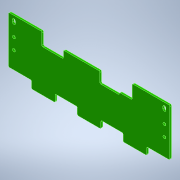
# Autodesk Inventor part: USB_MAIN_PCB
Saved by Autodesk Inventor 2021 (Build 250183000, 183)
## iProperties
Created: 2020-06-13
Part Number: USB_MAIN_PCB
Material: Generic
Document SubType Name: Modeling
Designer: Viktor Lindström
Density: 1 g/cm^3
Appearance: Default
Author: Viktor Lindström
Autodesk Inventor part; units mm, degrees
ref_plane "YZ Plane" through (0, 0, 0) normal (1, 0, 0) x (0, 1, 0)
ref_plane "XZ Plane" through (0, 0, 0) normal (0, 1, 0) x (-1, 0, 0)
ref_plane "XY Plane" through (0, 0, 0) normal (0, 0, 1) x (1, 0, 0)
sketch "Sketch1" plane through (0, 0, 0) normal (0, 0, 1) x (1, 0, 0)
  line L0 (-71, -23) -> (71, -23)
  line L1 (71, -23) -> (71, 23)
  line L2 (71, 23) -> (-71, 23)
  line L3 (-71, 23) -> (-71, -23)
  line L4 (-71, -23) -> (71, 23) construction
  line L5 (71, -23) -> (-71, 23) construction
  point P0 (0, 0)
  dimension "d2" = 142
  dimension "d3" = 46
  constraints: 12 end point, 2 midpoint, 2 parallel, 1 horizontal, 1 perpendicular
  measures "d2" distance of L1.end L2.end
  measures "d3" distance of L2.end L0.start
extrude "Extrusion1" add sketch "Sketch1" along normal blind 1.6
sketch "Sketch2" plane through (0, 0, 1.6) normal (0, 0, 1) x (1, 0, 0)
  line L0 (71, -23) -> (71, 23) projected
  line L1 (71, 23) -> (-71, 23) projected
  line L2 (-71, 23) -> (-71, -23) projected
  line L3 (-71, -23) -> (71, -23) projected
  line L4 (28, 23) -> (10, 23)
  line L5 (10, 23) -> (10, 13)
  line L6 (10, 13) -> (28, 13)
  line L7 (28, 13) -> (28, 23)
  point P0 (0, 0)
  dimension "d4" = 43
  dimension "d5" = 18
  dimension "d6" = 10
  constraints: 8 end point, 2 parallel, 1 horizontal, 1 perpendicular, 1 point on line
  measures "d4" distance between parallel lines of L7 L0
  measures "d5" distance between parallel lines of L7 L5
  measures "d6" distance between parallel lines of L1 L6
extrude "Extrusion2" cut sketch "Sketch2" against normal through all contours L7 L6 L5 L1
sketch "Sketch3" plane through (0, 0, 1.6) normal (0, 0, 1) x (1, 0, 0)
  line L0 (10, 13) -> (10, 23) construction
  line L1 (10, 23) -> (-71, 23) construction
  line L2 (-71, 23) -> (-71, -23) construction
  line L3 (-71, -23) -> (71, -23) construction
  line L4 (71, -23) -> (71, 23) construction
  line L5 (71, 23) -> (28, 23) construction
  line L6 (28, 23) -> (28, 13) construction
  line L7 (28, 13) -> (10, 13) construction
  line L8 (71, -23) -> (71, 23) projected
  line L9 (71, -23) -> (53.584, -23)
  line L10 (53.584, -23) -> (53.584, -16)
  line L11 (53.584, -16) -> (71, -16)
  line L12 (71, -16) -> (71, -23)
  line L13 (31.584, -23) -> (11, -23)
  line L14 (11, -23) -> (11, -16)
  line L15 (11, -16) -> (31.584, -16)
  line L16 (31.584, -16) -> (31.584, -23)
  line L17 (-71, -23) -> (71, -23) projected
  line L18 (-11, -23) -> (-31.584, -23)
  line L19 (-31.584, -23) -> (-31.584, -16)
  line L20 (-31.584, -16) -> (-11, -16)
  line L21 (-11, -16) -> (-11, -23)
  line L22 (-71, -23) -> (-53.584, -23)
  line L23 (-53.584, -23) -> (-53.584, -16)
  line L24 (-53.584, -16) -> (-71, -16)
  line L25 (-71, -16) -> (-71, -23)
  point P0 (0, 0)
  point P1 (3, -23)
  point P2 (-3, -23)
  dimension "d10" = 7
  dimension "d11" = 7
  dimension "d15" = 7
  dimension "d62" = 22
  dimension "d63" = 22
  dimension "d82" = 53.584
  dimension "d83" = 53.584
  dimension "d84" = 22
  dimension "d85" = 11
  constraints: 32 end point, 8 parallel, 4 horizontal, 4 perpendicular, 4 point on line
  measures "d10" distance between parallel lines of L22 L24
  measures "d11" distance between parallel lines of L9 L11
  measures "d15" distance between parallel lines of L13 L15
  measures "d62" distance between parallel lines of L19 L23
  measures "d63" distance between parallel lines of L10 L16
  measures "d82" distance from line of point (0, 0) L10
  measures "d83" distance from line of point (0, 0) L23
  measures "d84" distance between parallel lines of L21 L14
  measures "d85" distance from line of point (0, 0) L14
extrude "Extrusion3" cut sketch "Sketch3" against normal through all
sketch "Sketch5" plane through (0, 0, 1.6) normal (0, 0, 1) x (1, 0, 0)
  line L0 (-71, -16) -> (-53.584, -16) construction
  line L1 (53.584, -16) -> (71, -16) projected
  line L2 (-71, 23) -> (-71, -16) projected
  line L3 (-71, -16) -> (-75, -16)
  line L4 (-75, -16) -> (-75, 23)
  line L5 (-75, 23) -> (-71, 23)
  line L6 (-71, 23) -> (-71, -16)
  line L7 (71, 20) -> (71, -16)
  line L8 (0, -33.4899) -> (0, 38.4899) projected
  line L9 (71, 23) -> (71, -16)
  line L10 (71, -16) -> (75, -16)
  line L11 (75, -16) -> (75, 23)
  line L12 (75, 23) -> (71, 23)
  line L13 (71, 23) -> (71, -16)
  point P0 (0, 0)
  point P1 (71, 23)
  point P2 (71, 23)
  point P3 (-71, 22.2558)
  dimension "d32" = 75
  constraints: 20 end point, 4 symmetric about line, 2 parallel, 1 horizontal, 1 perpendicular, 1 point on line
  measures "d32" distance from line of L4 point (0, 0)
extrude "Extrusion5" add sketch "Sketch5" against normal up to surface (1.6 mm away)
sketch "Sketch6" plane through (0, 0, 0) normal (0, 0, -1) x (-1, 0, 0)
  circle A0 centre (70, 10.5) radius 1.375
  circle A1 centre (70, 0) radius 1.375
  line L0 (75, -16) -> (75, 23) construction
  line L1 (-10, 23) -> (75, 23) construction
  line L2 (0, -33.4899) -> (0, 38.4899) projected
  circle A2 centre (-70, 10.5) radius 1.375
  circle A3 centre (-70, 0) radius 1.375
  point P0 (0, 0)
  point P1 (-75, -16)
  point P2 (71, 23)
  dimension "d35" = 2.75
  dimension "d36" = 2.75
  dimension "d37" = 5
  dimension "d38" = 5
  dimension "d39" = 12.5
  dimension "d40" = 10.5
  constraints: 4 centre point, 3 symmetric about line, 2 other
  measures "d35" diameter of A1
  measures "d36" diameter of A0
  measures "d37" distance from line of L0 A1.centre
  measures "d38" distance from line of L0 A0.centre
  measures "d39" distance from line of L1 A0.centre
  measures "d40" distance of A0.centre A1.centre
extrude "Extrusion6" cut sketch "Sketch6" against normal through all
sketch "Sketch7" plane through (0, 0, 0) normal (0, 0, -1) x (-1, 0, 0)
  line L0 (-10, 23) -> (71, 23) projected
  line L1 (75, 23) -> (44, 23)
  line L2 (44, 23) -> (44, 28)
  line L3 (44, 28) -> (75, 28)
  line L4 (75, 28) -> (75, 23)
  line L5 (-75, 23) -> (-28, 23)
  line L6 (-28, 23) -> (-28, 28)
  line L7 (-28, 28) -> (-75, 28)
  line L8 (-75, 28) -> (-75, 23)
  point P0 (0, 0)
  dimension "d43" = 31
  dimension "d44" = 5
  dimension "d45" = 5
  constraints: 16 end point, 4 parallel, 2 horizontal, 2 perpendicular, 1 coincident
  measures "d43" distance between parallel lines of L4 L2
  measures "d44" distance between parallel lines of L0 L3
  measures "d45" distance between parallel lines of L5 L7
extrude "Extrusion7" add sketch "Sketch7" against normal up to surface (1.6 mm away)
sketch "Sketch8" plane through (0, 0, 0) normal (0, 0, -1) x (-1, 0, 0)
  circle A0 centre (70, 23) radius 1.375
  circle A1 centre (-70, 23) radius 1.375
  line L0 (75, -16) -> (75, 28) projected
  line L1 (75, 28) -> (44, 28) projected
  line L2 (-75, 28) -> (-75, -16) projected
  line L3 (-28, 28) -> (-75, 28) projected
  point P0 (0, 0)
  point P1 (75, 23)
  point P2 (-75, 23)
  dimension "d48" = 2.75
  dimension "d49" = 2.75
  dimension "d50" = 5
  dimension "d51" = 5
  dimension "d52" = 5
  dimension "d53" = 5
  constraints: 2 centre point
  measures "d48" diameter of A0
  measures "d49" diameter of A1
  measures "d50" distance from line of L0 A0.centre
  measures "d51" distance from line of L1 A0.centre
  measures "d52" distance from line of L2 A1.centre
  measures "d53" distance from line of L3 A1.centre
extrude "Extrusion8" cut sketch "Sketch8" against normal through all
fillet "Fillet1" radius 1 22 edges at (-75, 28, 0.8) (-75, -16, 0.8) (-53.584, -16, 0.8) (-53.584, -23, 0.8) (-31.584, -23, 0.8) (-11, -23, 0.8) (-11, -16, 0.8) (-31.584, -16, 0.8) (53.584, -16, 0.8) (53.584, -23, 0.8) (31.584, -23, 0.8) (31.584, -16, 0.8) (11, -23, 0.8) (11, -16, 0.8) (75, -16, 0.8) (75, 28, 0.8) (28, 28, 0.8) (28, 13, 0.8) (10, 13, 0.8) (10, 23, 0.8) (-44, 23, 0.8) (-44, 28, 0.8)
sketch "Sketch12" plane through (0, 0, 0) normal (0, 0, -1) x (-1, 0, 0)
  line L0 (-9, 23) -> (43, 23) projected
  line L1 (44, 27) -> (44, 24) projected
  line L2 (24, 16) -> (44, 16)
  line L3 (44, 16) -> (44, 24)
  line L4 (44, 24) -> (24, 24)
  line L5 (24, 24) -> (24, 16)
  line L6 (74, 28) -> (45, 28) projected
  point P0 (0, 0)
  dimension "d64" = 12
  dimension "d65" = 20
  constraints: 8 end point, 2 parallel, 1 horizontal, 1 perpendicular
  measures "d64" distance between parallel lines of L6 L2
  measures "d65" distance between parallel lines of L5 L3
extrude "Extrusion10" cut sketch "Sketch12" against normal through all
fillet "Fillet2" radius 1 3 edges at (-24, 23, 0.8) (-24, 16, 0.8) (-44, 16, 0.8)
sketch "Sketch13" plane through (0, 0, 0) normal (0, 0, -1) x (-1, 0, 0)
  line L0 (-29, 28) -> (-74, 28) projected
  line L1 (-27, 15) -> (-40, 15)
  line L2 (-40, 15) -> (-40, 28)
  line L3 (-40, 28) -> (-27, 28)
  line L4 (-27, 28) -> (-27, 15)
  line L5 (-28, 14) -> (-28, 27) projected
  point P0 (0, 0)
  point P1 (-27, 13)
  dimension "d74" = 13
  dimension "d75" = 12
  dimension "d76" = 0
  constraints: 8 end point, 2 parallel, 1 horizontal, 1 perpendicular, 1 point on line
  measures "d74" distance between parallel lines of L0 L1
  measures "d75" distance between parallel lines of L5 L2
  measures "d76" distance from line of point (-27, 13) L4
extrude "Extrusion11" cut sketch "Sketch13" against normal through all
fillet "Fillet3" radius 1 3 edges at (40, 15, 0.8) (40, 28, 0.8) (28, 15, 0.8)
sketch "Sketch14" plane through (0, 0, 0) normal (0, 0, -1) x (-1, 0, 0)
  line L0 (70, 24) -> (70, 22) construction
  line L1 (68.625, 24) -> (68.625, 22)
  line L2 (71.375, 22) -> (71.375, 24)
  arc A0 (71.375, 24) -> (68.625, 24) centre (70, 24) ccw
  arc A1 (68.625, 22) -> (71.375, 22) centre (70, 22) ccw
  circle A2 centre (70, 23) radius 1.375 projected
  line L3 (0, -33.4899) -> (0, 38.4899) projected
  line L4 (-70, 24) -> (-70, 22) construction
  line L5 (-68.625, 24) -> (-68.625, 22)
  line L6 (-71.375, 22) -> (-71.375, 24)
  arc A3 (-68.625, 24) -> (-71.375, 24) centre (-70, 24) ccw
  arc A4 (-71.375, 22) -> (-68.625, 22) centre (-70, 22) ccw
  circle A5 centre (-70, 23) radius 1.375
  point P0 (0, 0)
  point P1 (-70, 23)
  point P2 (68.625, 23)
  point P3 (71.375, 23)
  point P4 (-68.625, 23)
  point P5 (-71.375, 23)
  dimension "d81" = 2
  constraints: 16 end point, 8 point on circle, 8 symmetric about line, 5 centre point, 5 tangent, 1 midpoint, 1 parallel, 1 vertical, 3 other
  measures "d81" distance of L2.start L2.end
extrude "Extrusion12" cut sketch "Sketch14" against normal through all contours A0 L2 A2 L1 | A2 L2 A1 L1 | L5 A5 L6 A3 | L5 A4 L6 A5
sketch "FP_PCB_OUTLINE" plane through (0, 0, 1.6) normal (0, 0, 1) x (1, 0, 0)
  arc A0 (-44, 27) -> (-45, 28) centre (-45, 27) ccw projected
  line L0 (-74, 28) -> (-45, 28) projected
  arc A1 (-74, 28) -> (-75, 27) centre (-74, 27) ccw projected
  line L1 (-75, 27) -> (-75, -15) projected
  line L2 (-74, -16) -> (-54.584, -16) projected
  arc A2 (-53.584, -17) -> (-54.584, -16) centre (-54.584, -17) ccw projected
  line L3 (-53.584, -17) -> (-53.584, -22) projected
  arc A3 (-53.584, -22) -> (-52.584, -23) centre (-52.584, -22) ccw projected
  line L4 (-52.584, -23) -> (-32.584, -23) projected
  arc A4 (-32.584, -23) -> (-31.584, -22) centre (-32.584, -22) ccw projected
  line L5 (-31.584, -22) -> (-31.584, -17) projected
  arc A5 (-30.584, -16) -> (-31.584, -17) centre (-30.584, -17) ccw projected
  line L6 (-30.584, -16) -> (-12, -16) projected
  arc A6 (-11, -17) -> (-12, -16) centre (-12, -17) ccw projected
  line L7 (-11, -17) -> (-11, -22) projected
  arc A7 (-11, -22) -> (-10, -23) centre (-10, -22) ccw projected
  line L8 (-10, -23) -> (10, -23) projected
  arc A8 (10, -23) -> (11, -22) centre (10, -22) ccw projected
  line L9 (11, -22) -> (11, -17) projected
  arc A9 (12, -16) -> (11, -17) centre (12, -17) ccw projected
  line L10 (12, -16) -> (30.584, -16) projected
  arc A10 (31.584, -17) -> (30.584, -16) centre (30.584, -17) ccw projected
  line L11 (31.584, -17) -> (31.584, -22) projected
  arc A11 (31.584, -22) -> (32.584, -23) centre (32.584, -22) ccw projected
  line L12 (32.584, -23) -> (52.584, -23) projected
  arc A12 (52.584, -23) -> (53.584, -22) centre (52.584, -22) ccw projected
  line L13 (53.584, -22) -> (53.584, -17) projected
  arc A13 (54.584, -16) -> (53.584, -17) centre (54.584, -17) ccw projected
  line L14 (54.584, -16) -> (74, -16) projected
  line L15 (75, -15) -> (75, 27) projected
  arc A14 (75, 27) -> (74, 28) centre (74, 27) ccw projected
  line L16 (41, 28) -> (74, 28) projected
  arc A15 (27, 13) -> (28, 14) centre (27, 14) ccw projected
  line L17 (27, 13) -> (11, 13) projected
  arc A16 (10, 14) -> (11, 13) centre (11, 14) ccw projected
  line L18 (10, 14) -> (10, 22) projected
  arc A17 (10, 22) -> (9, 23) centre (9, 22) ccw projected
  line L19 (9, 23) -> (-23, 23) projected
  line L20 (-44, 27) -> (-44, 17) projected
  circle A18 centre (70, 0) radius 1.375 projected
  circle A19 centre (-70, 10.5) radius 1.375 projected
  circle A20 centre (70, 10.5) radius 1.375 projected
  circle A21 centre (-70, 0) radius 1.375 projected
  line L21 (2.354, 7.753) -> (2.354, 7.245) projected
  line L22 (2.354, 7.245) -> (1.846, 7.245) projected
  line L23 (1.846, 7.245) -> (1.846, 7.753) projected
  line L24 (1.846, 7.753) -> (2.354, 7.753) projected
  line L25 (-15.646, 9.245) -> (-16.154, 9.245) projected
  line L26 (-16.154, 9.753) -> (-15.646, 9.753) projected
  line L27 (-16.154, 9.245) -> (-16.154, 9.753) projected
  line L28 (-15.646, 9.753) -> (-15.646, 9.245) projected
  line L29 (-21.4, 21.25) -> (-21.4, 19.65) projected
  line L30 (-21.1, 19.65) -> (-21.1, 21.25) projected
  line L31 (-21.4, 19.45) -> (-21.1, 19.45) projected
  line L32 (-21.1, 21.45) -> (-21.4, 21.45) projected
  line L33 (-9.7, 19.45) -> (-9.4, 19.45) projected
  line L34 (-9.4, 19.65) -> (-9.4, 21.25) projected
  line L35 (-9.7, 21.25) -> (-9.7, 19.65) projected
  line L36 (-9.4, 21.45) -> (-9.7, 21.45) projected
  line L37 (-4.4, 21.25) -> (-4.4, 19.65) projected
  line L38 (-4.4, 19.45) -> (-4.1, 19.45) projected
  line L39 (-4.1, 19.65) -> (-4.1, 21.25) projected
  line L40 (-4.1, 21.45) -> (-4.4, 21.45) projected
  line L41 (7.3, 19.45) -> (7.6, 19.45) projected
  line L42 (7.6, 19.65) -> (7.6, 21.25) projected
  line L43 (7.3, 21.25) -> (7.3, 19.65) projected
  line L44 (7.6, 21.45) -> (7.3, 21.45) projected
  line L45 (5.5, 17.55) -> (5.7, 17.55) projected
  line L46 (-2.5, 17.55) -> (-2.3, 17.55) projected
  line L47 (-2.6, 18.7526) -> (-2.6, 17.65) projected
  line L48 (5.8, 18.7526) -> (5.8, 17.65) projected
  line L49 (-11.2, 18.7526) -> (-11.2, 17.65) projected
  line L50 (-11.5, 17.55) -> (-11.3, 17.55) projected
  line L51 (-19.5, 17.55) -> (-19.3, 17.55) projected
  line L52 (-19.6, 18.7526) -> (-19.6, 17.65) projected
  line L53 (-20.8, 23.5) -> (-15.415, 23.5) projected
  line L54 (1.615, 23.5) -> (7, 23.5) projected
  line L55 (-3.8, 23.5) -> (1.585, 23.5) projected
  line L56 (-15.385, 23.5) -> (-10, 23.5) projected
  circle A22 centre (2.1, 7.499) radius 0.3592
  circle A23 centre (-15.9, 9.499) radius 0.3592
  circle A24 centre (-21.25, 20.45) radius 1
  circle A25 centre (-9.55, 20.45) radius 1
  circle A26 centre (-4.25, 20.45) radius 1
  circle A27 centre (7.45, 20.45) radius 1
  arc A28 (29, 15) -> (28, 14) centre (29, 14) ccw projected
  arc A29 (-23, 23) -> (-24, 22) centre (-23, 22) ccw projected
  line L57 (-24, 22) -> (-24, 17) projected
  arc A30 (-25, 16) -> (-24, 17) centre (-25, 17) ccw projected
  line L58 (-25, 16) -> (-43, 16) projected
  arc A31 (-44, 17) -> (-43, 16) centre (-43, 17) ccw projected
  arc A32 (41, 28) -> (40, 27) centre (41, 27) ccw projected
  line L59 (40, 27) -> (40, 16) projected
  arc A33 (39, 15) -> (40, 16) centre (39, 16) ccw projected
  line L60 (39, 15) -> (29, 15) projected
  arc A34 (-75, -15) -> (-74, -16) centre (-74, -15) ccw projected
  arc A35 (74, -16) -> (75, -15) centre (74, -15) ccw projected
  arc A36 (71.375, 24) -> (68.625, 24) centre (70, 24) ccw projected
  line L61 (71.375, 22) -> (71.375, 24) projected
  arc A37 (68.625, 22) -> (71.375, 22) centre (70, 22) ccw projected
  line L62 (68.625, 24) -> (68.625, 22) projected
  arc A38 (-68.625, 24) -> (-71.375, 24) centre (-70, 24) ccw projected
  line L63 (-68.625, 22) -> (-68.625, 24) projected
  arc A39 (-71.375, 22) -> (-68.625, 22) centre (-70, 22) ccw projected
  line L64 (-71.375, 24) -> (-71.375, 22) projected
  circle A40 centre (-51.35, 10.5) radius 0.7937
  circle A41 centre (-38.65, 10.5) radius 0.7937
  circle A42 centre (-51.35, 0) radius 0.7937
  circle A43 centre (-38.65, 0) radius 0.7937
  circle A44 centre (51.35, 0) radius 0.7937
  circle A45 centre (51.35, 10.5) radius 0.7937
  circle A46 centre (38.65, 10.5) radius 0.7937
  circle A47 centre (38.65, 0) radius 0.7937
  line L65 (49.154, -13.9809) -> (48.3188, -14.7)
  line L66 (49.154, -13.9809) -> (48.3188, -14.7)
  line L67 (49.154, -13.9809) -> (49.9892, -14.7)
  line L68 (49.9892, -14.7) -> (49.154, -15.4191)
  line L69 (49.154, -15.4191) -> (48.3188, -14.7)
  line L70 (49.184, -18.3309) -> (48.3488, -19.05)
  line L71 (50.0192, -19.05) -> (49.184, -18.3309)
  line L72 (49.184, -19.7691) -> (50.0192, -19.05)
  line L73 (48.3488, -19.05) -> (49.184, -19.7691)
  line L74 (35.984, -19.8852) -> (36.7031, -19.05)
  line L75 (36.7031, -19.05) -> (35.984, -18.2148)
  line L76 (35.984, -18.2148) -> (35.2649, -19.05)
  line L77 (35.2649, -19.05) -> (35.984, -19.8852)
  line L78 (36.014, -15.5352) -> (36.7331, -14.7)
  line L79 (36.014, -13.8648) -> (36.7331, -14.7)
  line L80 (35.2949, -14.7) -> (36.014, -13.8648)
  line L81 (36.014, -15.5352) -> (35.2949, -14.7)
  line L82 (6.57, -15.4191) -> (5.7348, -14.7)
  line L83 (6.57, -13.9809) -> (5.7348, -14.7)
  line L84 (6.57, -13.9809) -> (7.4052, -14.7)
  line L85 (7.4052, -14.7) -> (6.57, -15.4191)
  line L86 (-6.57, -15.5352) -> (-5.8509, -14.7)
  line L87 (-6.57, -13.8648) -> (-5.8509, -14.7)
  line L88 (-7.2891, -14.7) -> (-6.57, -13.8648)
  line L89 (-6.57, -15.5352) -> (-7.2891, -14.7)
  line L90 (-35.1788, -14.7) -> (-36.014, -15.4191)
  line L91 (-36.014, -13.9809) -> (-35.1788, -14.7)
  line L92 (-36.014, -13.9809) -> (-36.8492, -14.7)
  line L93 (-36.014, -15.4191) -> (-36.8492, -14.7)
  line L94 (-49.154, -15.5352) -> (-48.4349, -14.7)
  line L95 (-49.154, -13.8648) -> (-48.4349, -14.7)
  line L96 (-49.8731, -14.7) -> (-49.154, -13.8648)
  line L97 (-49.154, -15.5352) -> (-49.8731, -14.7)
  circle A48 centre (36.014, -14.7) radius 0.8352
  circle A49 centre (49.154, -14.7) radius 0.7191
  circle A50 centre (49.184, -19.05) radius 0.7191
  circle A51 centre (35.984, -19.05) radius 0.8352
  circle A52 centre (-6.57, -14.7) radius 0.8352
  circle A53 centre (6.57, -14.7) radius 0.7191
  circle A54 centre (-36.014, -14.7) radius 0.7191
  circle A55 centre (-49.154, -14.7) radius 0.8352
  point P0 (0, 0)
  point P1 (-21.5726, -14.5695)
  constraints: 66 end point, 12 centre point, 8 vertical alignment, 104 other
equation "\"d11\" = d10"
equation "\"d15\" = d11"
equation "\"d63\" = d62"
equation "\"d36\" = d35"
equation "\"d45\" = d44"
equation "\"d49\" = d48"
equation "\"d51\" = d50"
equation "\"d52\" = d50"
equation "\"d53\" = d52"
body "Solid1"
